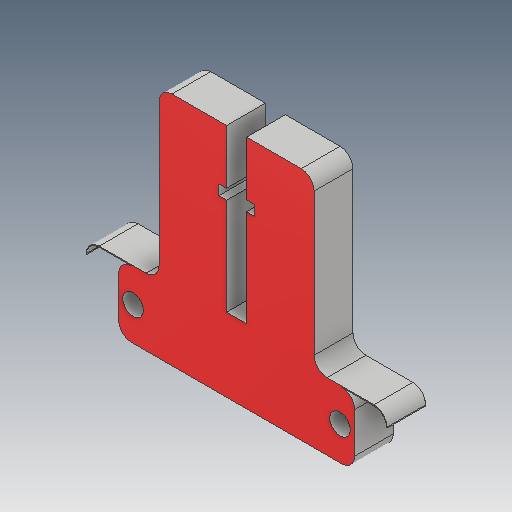
# Autodesk Inventor part: Hotend Slide Part 1
Saved by Autodesk Inventor 2017 (Build 210142000, 142)
## iProperties
Created: 2016-06-24
Part Number: Hotend Slide Part 1
Material: Generic
Document SubType Name: Modeling
Designer: joshm
Density: 1 g/cm^3
Appearance: Default
Mass: 5.4107 g
Surface Area: 30.8482 cm^2
Volume: 5.4107 cm^3
Author: joshm
Autodesk Inventor part; units mm, degrees
ref_plane "YZ Plane" through (0, 0, 0) normal (1, 0, 0) x (0, 1, 0)
ref_plane "XZ Plane" through (0, 0, 0) normal (0, 1, 0) x (-1, 0, 0)
ref_plane "XY Plane" through (0, 0, 0) normal (0, 0, 1) x (1, 0, 0)
sketch "Sketch1" plane through (0, 0, 0) normal (0, 0, 1) x (1, 0, 0)
  line L0 (-21.2294, -12.5998) -> (21.2706, -12.5998)
  line L1 (23.2706, -10.5998) -> (23.2706, -4.1998)
  line L2 (-23.2294, -4.1998) -> (-23.2294, -10.5998)
  line L3 (12.0206, -0.1998) -> (12.0206, 21.8002)
  line L4 (10.0206, 23.8002) -> (-9.9794, 23.8002)
  line L5 (-11.9794, 21.8002) -> (-11.9794, -0.1998)
  circle A0 centre (16.0206, -7.3998) radius 1.6
  circle A1 centre (-15.9794, -7.3998) radius 1.6
  line L6 (21.2706, -2.1998) -> (14.0206, -2.1998)
  line L7 (-13.9794, -2.1998) -> (-21.2294, -2.1998)
  line L8 (0.0206, 11.8002) -> (-1.5294, 11.8002)
  line L9 (-1.5294, 11.8002) -> (1.5706, 11.8002)
  line L10 (-1.5294, 11.8002) -> (-1.5294, 13.8002)
  line L11 (-1.5294, 13.8002) -> (-2.7282, 13.8002)
  line L12 (2.7718, 13.8002) -> (2.7718, 15.8002)
  line L13 (-2.7282, 15.8002) -> (-2.7282, 13.8002)
  line L14 (-2.7282, 15.8002) -> (-1.5294, 15.8002)
  line L15 (0.0206, 15.8002) -> (0.0218, 15.8002)
  line L16 (2.7718, 15.8002) -> (1.5706, 15.8002)
  line L17 (-1.5294, 15.8002) -> (-2.7282, 15.8002)
  line L18 (-1.5294, 11.8002) -> (-1.5294, 13.8002)
  line L19 (-1.5294, 15.8002) -> (-1.5294, 23.8002)
  line L20 (-2.7282, 13.8002) -> (-1.5294, 13.8002)
  line L21 (1.5706, 13.8002) -> (2.7718, 13.8002)
  line L22 (1.5706, 11.8002) -> (1.5706, 13.8002)
  line L23 (1.5706, 15.8002) -> (1.5706, 23.8002)
  arc A2 (23.2706, -4.1998) -> (21.2706, -2.1998) centre (21.2706, -4.1998) ccw
  arc A3 (21.2706, -12.5998) -> (23.2706, -10.5998) centre (21.2706, -10.5998) ccw
  arc A4 (-23.2294, -10.5998) -> (-21.2294, -12.5998) centre (-21.2294, -10.5998) ccw
  arc A5 (-21.2294, -2.1998) -> (-23.2294, -4.1998) centre (-21.2294, -4.1998) ccw
  arc A6 (-13.9794, -2.1998) -> (-11.9794, -0.1998) centre (-13.9794, -0.1998) ccw
  arc A7 (12.0206, -0.1998) -> (14.0206, -2.1998) centre (14.0206, -0.1998) ccw
  arc A8 (-9.9794, 23.8002) -> (-11.9794, 21.8002) centre (-9.9794, 21.8002) ccw
  arc A9 (12.0206, 21.8002) -> (10.0206, 23.8002) centre (10.0206, 21.8002) ccw
  point P0 (0, 0)
  point P1 (0, 0)
  point P2 (12.0206, 23.8002)
  point P3 (-11.9794, 23.8002)
  dimension "d0" = 24
  dimension "d1" = 3.2
  dimension "d2" = 3.2
  dimension "d3" = 2
  constraints: 48 end point, 16 point on circle, 16 tangent, 10 centre point, 9 parallel, 8 perpendicular, 7 equal radius, 7 point on line, 3 horizontal
  measures "d0" distance of point (-11.979, 23.8) point (12.021, 23.8)
  measures "d1" diameter of A0
  measures "d2" diameter of A1
  measures "d3" radius of A2
extrude "Extrusion1" add sketch "Sketch1" along normal blind 6 contours A4 L2 A5 L7 A6 L5 A8 L4 L19 L14 L13 L11 L10 L8 L9 L22 L21 L12 L16 L23 A9 L3 A7 L6 A2 L1 A3 L0
sketch "Sketch2" plane through (0, 0, 6) normal (0, 0, 1) x (1, 0, 0)
  circle A0 centre (-6.9812, 28.6469) radius 1.6
  circle A1 centre (7.0188, 28.6469) radius 1.6
  circle A2 centre (-17.6062, 13.3479) radius 1.6
  circle A3 centre (17.6438, 13.3479) radius 1.6
  line L0 (-23.2312, 26.8921) -> (-23.2312, -30.3531)
  arc A4 (-23.2312, -30.3531) -> (-21.2312, -32.3531) centre (-21.2312, -30.3531) ccw
  line L1 (-21.2312, -32.3531) -> (-7.8931, -32.3531)
  arc A5 (21.2688, -32.3531) -> (23.2688, -30.3531) centre (21.2688, -30.3531) ccw
  line L2 (23.2688, -30.3531) -> (23.2688, 26.8921)
  arc A6 (23.2688, 26.8921) -> (21.8599, 27.8047) centre (22.2688, 26.8921) ccw
  arc A7 (12.0188, 33.6469) -> (21.8599, 27.8047) centre (18.9975, 34.1927) ccw
  line L3 (12.0188, 33.6469) -> (12.0188, 39.5469)
  arc A8 (12.0188, 39.5469) -> (10.0188, 41.5469) centre (10.0188, 39.5469) ccw
  line L4 (10.0188, 41.5469) -> (2.5188, 41.5469)
  arc A9 (2.5188, 41.5469) -> (1.5188, 40.5469) centre (2.5188, 40.5469) ccw
  line L5 (1.5188, 40.5469) -> (1.5188, 36.5469)
  line L6 (1.5188, 36.5469) -> (2.7688, 36.5469)
  line L7 (2.7688, 36.5469) -> (2.7688, 33.6469)
  line L8 (2.7688, 33.6469) -> (1.5688, 33.6469)
  line L9 (1.5688, 33.6469) -> (1.5688, 23.6469)
  line L10 (1.5688, 23.6469) -> (10.0188, 23.6469)
  arc A10 (12.0188, 21.6469) -> (10.0188, 23.6469) centre (10.0188, 21.6469) ccw
  line L11 (12.0188, 21.6469) -> (12.0188, -0.3531)
  arc A11 (12.0188, -0.3531) -> (14.0188, -2.3531) centre (14.0188, -0.3531) ccw
  line L12 (14.0206, -2.3531) -> (16.2688, -2.3531)
  arc A12 (18.2688, -4.3531) -> (16.2688, -2.3531) centre (16.2688, -4.3531) ccw
  line L13 (18.2688, -4.3531) -> (18.2688, -21.3531)
  arc A13 (16.2688, -23.3531) -> (18.2688, -21.3531) centre (16.2688, -21.3531) ccw
  line L14 (16.2688, -23.3531) -> (-16.2312, -23.3531)
  arc A14 (-18.2312, -21.3531) -> (-16.2312, -23.3531) centre (-16.2312, -21.3531) ccw
  line L15 (-18.2312, -21.3531) -> (-18.2312, -4.3531)
  arc A15 (-16.2312, -2.3531) -> (-18.2312, -4.3531) centre (-16.2312, -4.3531) ccw
  line L16 (-16.2312, -2.3531) -> (-13.9794, -2.3531)
  arc A16 (-13.9794, -2.3531) -> (-11.9812, -0.5065) centre (-13.9753, -0.3531) ccw
  line L17 (-11.9812, -0.5065) -> (-11.9812, 21.4935)
  arc A17 (-9.9812, 23.4935) -> (-11.9812, 21.4935) centre (-9.9812, 21.4935) ccw
  line L18 (-9.9812, 23.4935) -> (-1.5312, 23.4935)
  line L19 (-1.5312, 23.4935) -> (-1.5312, 33.4935)
  line L20 (-1.5312, 33.4935) -> (-2.7312, 33.4935)
  line L21 (-2.7312, 33.4935) -> (-2.7312, 36.3935)
  line L22 (-2.7312, 36.3935) -> (-1.4812, 36.3935)
  line L23 (-1.4812, 36.3935) -> (-1.4812, 40.5469)
  arc A18 (-1.4812, 40.5469) -> (-2.4812, 41.5469) centre (-2.4812, 40.5469) ccw
  line L24 (-2.4812, 41.5469) -> (-9.9812, 41.5469)
  arc A19 (-9.9812, 41.5469) -> (-11.9812, 39.5469) centre (-9.9812, 39.5469) ccw
  line L25 (-11.9812, 39.5469) -> (-11.9812, 33.6469)
  arc A20 (-21.8223, 27.8047) -> (-11.9812, 33.6469) centre (-18.9599, 34.1927) ccw
  arc A21 (-21.8223, 27.8047) -> (-23.2312, 26.8921) centre (-22.2312, 26.8921) ccw
  line L26 (-13.9794, -2.3531) -> (-21.2294, -2.3531)
  arc A22 (-21.2294, -2.3531) -> (-23.2294, -4.3531) centre (-21.2294, -4.3531) ccw
  line L27 (-23.2294, -4.3531) -> (-23.2294, -10.7531)
  arc A23 (-23.2294, -10.7531) -> (-21.2294, -12.7531) centre (-21.2294, -10.7531) ccw
  line L28 (-21.2294, -12.7531) -> (21.2706, -12.7531)
  line L29 (21.2706, -2.3531) -> (14.0206, -2.3531)
  arc A24 (23.2706, -4.3531) -> (21.2706, -2.3531) centre (21.2706, -4.3531) ccw
  line L30 (23.2706, -10.7531) -> (23.2706, -4.3531)
  arc A25 (21.2706, -12.7531) -> (23.2706, -10.7531) centre (21.2706, -10.7531) ccw
  arc A26 (5.9613, -30.7014) -> (7.9307, -32.3531) centre (7.9307, -30.3531) ccw
  line L31 (7.9307, -32.3531) -> (21.2688, -32.3531)
  arc A27 (-7.8931, -32.3531) -> (-5.9236, -30.7014) centre (-7.8931, -30.3531) ccw
  arc A28 (5.9613, -30.7014) -> (-5.9236, -30.7014) centre (0.0188, -31.7522) ccw
  point P0 (0, 0)
  point P1 (-18.2312, -12.7531)
  point P2 (18.2688, -12.7531)
  constraints: 60 end point, 50 point on circle, 29 centre point, 4 point on line, 6 other
extrude "Extrusion2" cut sketch "Sketch2" against normal blind 6 contours A22 L26 A15 L15 L28 A23 L0 | L13 A12 L29 A24 L2 A25 L28
fillet "Fillet1" radius 2 2 edges at (18.2688, -12.5998, 3) (-18.2312, -12.5998, 3)
sketch "Sketch4" plane through (-1.5294, 11.8002, 0) normal (0, 1, 0) x (1, 0, 0)
  line L0 (3.1, 0) -> (0, 0) projected
  line L1 (0, 0) -> (0, -6) projected
  line L2 (3.1, -6) -> (0, -6) projected
  line L3 (3.1, 0) -> (3.1, -6) projected
  point P0 (1.5294, 0)
extrude "Extrusion3" cut sketch "Sketch4" against normal blind 13
sketch "Sketch5" plane through (-2.7282, 15.8002, 0) normal (0, -1, 0) x (1, 0, 0)
  line L0 (0, 0) -> (1.1988, 0) projected
  line L1 (1.1988, 0) -> (1.1988, 6) projected
  line L2 (0, 6) -> (1.1988, 6) projected
  line L3 (0, 0) -> (0, 6) projected
  line L4 (4.2988, 0) -> (5.5, 0) projected
  line L5 (5.5, 0) -> (5.5, 6) projected
  line L6 (4.2988, 6) -> (5.5, 6) projected
  line L7 (4.2988, 0) -> (4.2988, 6) projected
  point P0 (2.7282, 0)
extrude "Extrusion4" add sketch "Sketch5" along normal blind 0.4
sketch "Sketch6" plane through (0, 0, 6) normal (0, 0, 1) x (1, 0, 0)
  line L0 (22.9743, 18.6641) -> (86.0826, 18.6641) construction
  line L1 (86.0826, 18.6641) -> (86.0826, -0.0954) construction
  line L2 (86.0826, -0.0954) -> (22.9743, -0.0954) construction
  line L3 (22.9743, -0.0954) -> (22.9743, 18.6641) construction
  point P0 (0, 0)
  constraints: 2 other
extrude "Extrusion5" [suppressed]
body "Solid1"
